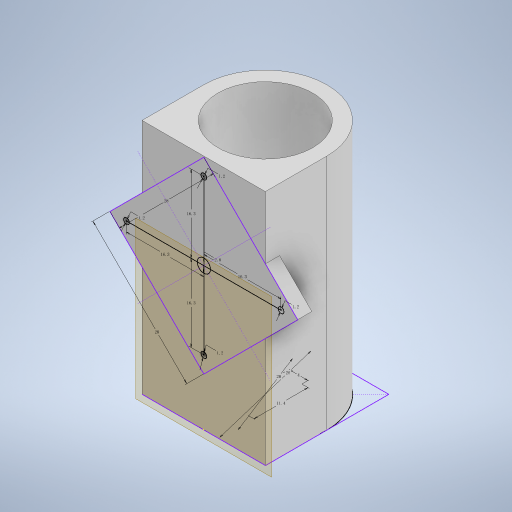
# Autodesk Inventor part: 固定件
Saved by Autodesk Inventor 2023 (Build 270158000, 158)
## iProperties
Created: 2022-10-17
Part Number: 固定件
Material: 常规
Document SubType Name: Sheet Metal
Designer: 22215
Density: 1 g/cm^3
Sheet Metal Rule: 默认_mm
Appearance: 默认
Author: 22215
Autodesk Inventor part; units mm, degrees
ref_plane "YZ Plane" through (0, 0, 0) normal (1, 0, 0) x (0, 1, 0)
ref_plane "XZ Plane" through (0, 0, 0) normal (0, 1, 0) x (-1, 0, 0)
sketch "草图1" plane through (0, 0, 0) normal (0, 1, 0) x (-1, 0, 0)
  circle A0 centre (0, 0) radius 10
  circle A1 centre (0, 0) radius 13
  line L0 (2, 5.7) -> (-2, 5.7)
  line L1 (-2, 5.7) -> (-2, -5.7)
  line L2 (-2, -5.7) -> (2, -5.7)
  line L3 (2, -5.7) -> (2, 5.7)
  line L4 (2, 5.7) -> (-2, -5.7) construction
  line L5 (-2, 5.7) -> (2, -5.7) construction
  line L6 (13, 13) -> (-13, 13)
  line L7 (-13, 13) -> (-13, -13)
  line L8 (-13, -13) -> (13, -13)
  line L9 (13, -13) -> (13, 13)
  line L10 (13, 13) -> (-13, -13) construction
  line L11 (-13, 13) -> (13, -13) construction
  point P0 (13, 0)
  point P1 (0, 13)
  point P2 (-13, 0)
  dimension "d0" = 20
  dimension "d1" = 26
  dimension "d2" = 4
  dimension "d3" = 11.4
  constraints: 24 end point, 4 midpoint, 4 parallel, 2 centre point, 2 coincident, 2 horizontal, 2 perpendicular
  measures "d0" diameter of A0
  measures "d1" diameter of A1
  measures "d2" distance of L2.end L1.end
  measures "d3" distance of L1.end L0.end
extrude "拉伸1" add sketch "草图1" along normal blind 12 contours A0
extrude "拉伸2" add sketch "草图1" along normal blind 30 contours A1
ref_plane "工作平面1" through (0, 0, 13) normal (0, 0, 1) x (1, 0, 0)
sketch "草图2" plane through (0, 0, 13) normal (0, 0, 1) x (1, 0, 0)
  line L0 (-10, 30) -> (10, 30) projected
  circle A0 centre (0, 30) radius 1.4
  line L1 (0, 30) -> (0, 46.3)
  line L2 (0, 30) -> (0, 13.7)
  circle A1 centre (0, 13.7) radius 0.6
  circle A2 centre (0, 46.3) radius 0.6
  line L3 (0, 30) -> (16.3, 30)
  line L4 (0, 30) -> (-16.3, 30)
  line L5 (13, 30) -> (-13, 30) projected
  circle A3 centre (16.3, 30) radius 0.6
  circle A4 centre (-16.3, 30) radius 0.6
  line L6 (19.799, 30) -> (0, 10.201)
  line L7 (0, 10.201) -> (-19.799, 30)
  line L8 (-19.799, 30) -> (0, 49.799)
  line L9 (0, 49.799) -> (19.799, 30)
  line L10 (-14, 44) -> (14, 16) construction
  line L11 (14, 44) -> (-14, 16) construction
  point P0 (0, 0)
  dimension "d9" = 2.8
  dimension "d10" = 16.3
  dimension "d11" = 16.3
  dimension "d12" = 1.2
  dimension "d13" = 1.2
  dimension "d14" = 16.3
  dimension "d15" = 16.3
  dimension "d16" = 1.2
  dimension "d17" = 1.2
  dimension "d20" = 28
  dimension "d21" = 28
  constraints: 20 end point, 5 centre point, 4 coincident, 3 midpoint, 2 parallel, 2 perpendicular, 1 collinear, 1 horizontal, 1 vertical
  measures "d9" diameter of A0
  measures "d10" distance of L1.start L1.end
  measures "d11" distance of L1.start L2.end
  measures "d12" diameter of A1
  measures "d13" diameter of A2
  measures "d14" distance of L1.start L3.end
  measures "d15" distance of L1.start L4.end
  measures "d16" diameter of A3
  measures "d17" diameter of A4
  measures "d20" distance of L7.end L8.end
  measures "d21" distance between parallel lines of L8 L6
extrude "拉伸3" add sketch "草图1" along normal blind 50 contours A1 | A1 L6 L9 | A1 L7 L6
extrude "拉伸4" add sketch "草图2" against normal blind 3
extrude "拉伸5" cut sketch "草图2" against normal blind 10 contours A2
extrude "拉伸6" cut sketch "草图2" against normal blind 10 contours A1
equation "\"折弯半径\" = 厚度"
equation "\"折弯释压宽度\" = 厚度"
equation "\"折弯释压深度\" = 0.5 * 厚度"
equation "\"拐角释压尺寸\" = 4 * 厚度"
equation "\"最小余量\" = 2 * 厚度"
equation "\"过渡半径\" = 折弯半径"
equation "\"Jacobi半径尺寸\" = 折弯半径"
equation "\"间隙大小\" = 厚度"
equation "\"厚度\" = 0.5"
